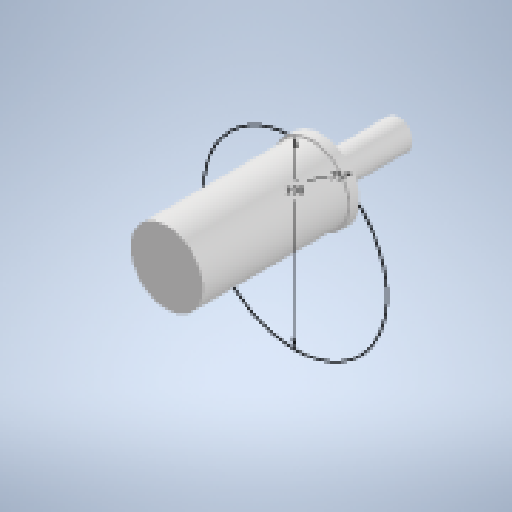
# Autodesk Inventor part: MotorPart2
Saved by Autodesk Inventor 2024 (Build 280153000, 153)
## iProperties
Created: 2024-10-17
Part Number: MotorPart2
Material: 一般
Document SubType Name: Modeling
Designer: jerry
Density: 1 g/cm^3
Appearance: 預設
Author: jerry
Autodesk Inventor part; units mm, degrees
ref_plane "YZ Plane" through (0, 0, 0) normal (1, 0, 0) x (0, 1, 0)
ref_plane "XZ Plane" through (0, 0, 0) normal (0, 1, 0) x (-1, 0, 0)
ref_plane "XY Plane" through (0, 0, 0) normal (0, 0, 1) x (1, 0, 0)
sketch "草圖1" plane through (0, 0, 0) normal (0, 0, 1) x (1, 0, 0)
  circle A0 centre (0, 0) radius 95
  circle A1 centre (27.5, 72) radius 37.5
  dimension "d0" = 190
  dimension "d3" = 75
  constraints: 2 centre point, 1 coincident
  measures "d0" diameter of A0
  measures "d3" diameter of A1
extrude "擠出1" add sketch "草圖1" along normal blind 160 contours A1 A0 | A0 A1 picked at (37.7638, 69.1742) picked at (30.5515, 96.5803)
sketch "草圖2" plane through (27.5, 72, 0) normal (0, 0, -1) x (-1, 0, 0)
  circle A0 centre (0, 0) radius 40
  point P0 (27.5, -72)
  dimension "d6" = 80
  constraints: 1 centre point
  measures "d6" diameter of A0
extrude "擠出2" add sketch "草圖2" against normal blind 10
sketch "草圖3" plane through (27.5, 72, 0) normal (0, 0, -1) x (-1, 0, 0)
  circle A0 centre (0, 0) radius 15
  point P0 (27.5, -72)
  dimension "d9" = 30
  constraints: 1 centre point
  measures "d9" diameter of A0
extrude "擠出3" add sketch "草圖3" along normal blind 80
